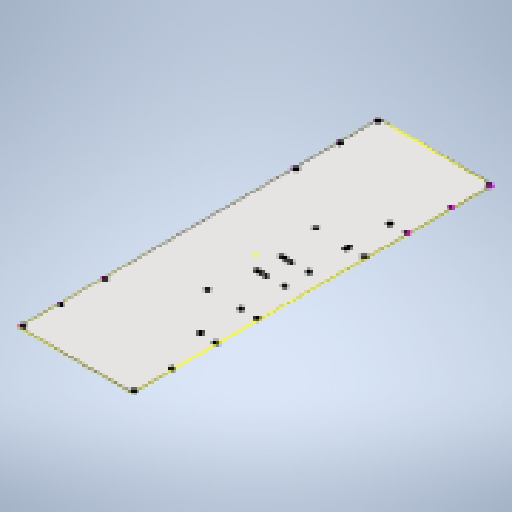
# Autodesk Inventor part: Base sheet2
Saved by Autodesk Inventor 2025.2 (Build 292293000, 293)
## iProperties
Created: 2025-05-26
Part Number: Base sheet2
Material: Generic
Document SubType Name: Sheet Metal
Designer: abdal
Density: 1 g/cm^3
Sheet Metal Rule: Default_mm
Appearance: Default
Author: abdal
Autodesk Inventor part; units mm, degrees
ref_plane "YZ Plane" through (0, 0, 0) normal (1, 0, 0) x (0, 1, 0)
ref_plane "XZ Plane" through (0, 0, 0) normal (0, 1, 0) x (-1, 0, 0)
ref_plane "XY Plane" through (0, 0, 0) normal (0, 0, 1) x (1, 0, 0)
sketch "Sketch1" plane through (0, 0, 0) normal (0, 1, 0) x (-1, 0, 0)
  line L0 (515, 1626) -> (-515, 1626)
  line L1 (-515, 1626) -> (-515, -1626)
  line L2 (-515, -1626) -> (515, -1626)
  line L3 (515, -1626) -> (515, 1626)
  line L4 (515, 1626) -> (-515, -1626) construction
  line L5 (-515, 1626) -> (515, -1626) construction
  point P0 (0, 0)
  dimension "d0" = 3252
  dimension "d1" = 1030
  measures "d0" distance of L2.end L0.start
  measures "d1" distance of L1.end L2.end
extrude "Plate1" add sketch "Sketch1" along normal blind 3
sketch "Sketch2" plane through (0, 0, 0) normal (0, -1, 0) x (1, 0, 0)
  line L0 (491, 1591.5799) -> (509, 1591.5799)
  ellipse E0 centre (509, 1594.777) end of major axis (509, 1597.9742) minor radius 3 (509, 1591.5799) -> (512, 1594.777) ccw
  line L1 (512, 1594.777) -> (512, 1613.9598)
  ellipse E1 centre (509, 1613.9598) end of major axis (509, 1610.7627) minor radius 3 (512, 1613.9598) -> (509, 1617.1569) ccw
  line L2 (509, 1617.1569) -> (491, 1617.1569)
  ellipse E2 centre (491, 1613.9598) end of major axis (491, 1610.7627) minor radius 3 (491, 1617.1569) -> (488, 1613.9598) ccw
  line L3 (488, 1613.9598) -> (488, 1594.777)
  ellipse E3 centre (491, 1594.777) end of major axis (491, 1597.9742) minor radius 3 (488, 1594.777) -> (491, 1591.5799) ccw
  line L4 (515, 1613.9598) -> (515, 1594.777)
  ellipse E4 centre (509, 1594.777) end of major axis (509, 1601.1713) minor radius 6 (509, 1588.3828) -> (515, 1594.777) ccw
  line L5 (509, 1588.3828) -> (491, 1588.3828)
  ellipse E5 centre (491, 1594.777) end of major axis (491, 1601.1713) minor radius 6 (485, 1594.777) -> (491, 1588.3828) ccw
  line L6 (485, 1594.777) -> (485, 1613.9598)
  ellipse E6 centre (491, 1613.9598) end of major axis (491, 1607.5655) minor radius 6 (491, 1620.354) -> (485, 1613.9598) ccw
  line L7 (491, 1620.354) -> (509, 1620.354)
  ellipse E7 centre (509, 1613.9598) end of major axis (509, 1607.5655) minor radius 6 (515, 1613.9598) -> (509, 1620.354) ccw
  line L8 (512, 1252) -> (512, 1270)
  arc A0 (512, 1270) -> (509, 1273) centre (509, 1270) ccw
  line L9 (509, 1273) -> (491, 1273)
  arc A1 (491, 1273) -> (488, 1270) centre (491, 1270) ccw
  line L10 (488, 1270) -> (488, 1252)
  arc A2 (488, 1252) -> (491, 1249) centre (491, 1252) ccw
  line L11 (491, 1249) -> (509, 1249)
  arc A3 (509, 1249) -> (512, 1252) centre (509, 1252) ccw
  line L12 (509, 1246) -> (491, 1246)
  arc A4 (485, 1252) -> (491, 1246) centre (491, 1252) ccw
  line L13 (485, 1252) -> (485, 1270)
  arc A5 (491, 1276) -> (485, 1270) centre (491, 1270) ccw
  line L14 (491, 1276) -> (509, 1276)
  arc A6 (515, 1270) -> (509, 1276) centre (509, 1270) ccw
  line L15 (515, 1270) -> (515, 1252)
  arc A7 (509, 1246) -> (515, 1252) centre (509, 1252) ccw
  line L16 (340.4848, 863.6493) -> (340.3575, 844.2981)
  ellipse E8 centre (343.3574, 844.2783) end of major axis (343.3787, 847.5035) minor radius 3 (340.3575, 844.2981) -> (343.3362, 841.0531) ccw
  line L17 (343.3362, 841.0531) -> (361.3358, 840.9347)
  ellipse E9 centre (361.3571, 844.1599) end of major axis (361.3783, 847.3851) minor radius 3 (361.3358, 840.9347) -> (364.357, 844.1401) ccw
  line L18 (364.357, 844.1401) -> (364.4843, 863.4914)
  ellipse E10 centre (361.4844, 863.5111) end of major axis (361.4632, 860.2859) minor radius 3 (364.4843, 863.4914) -> (361.5056, 866.7363) ccw
  line L19 (361.5056, 866.7363) -> (343.506, 866.8548)
  ellipse E11 centre (343.4848, 863.6296) end of major axis (343.4636, 860.4044) minor radius 3 (343.506, 866.8548) -> (340.4848, 863.6493) ccw
  ellipse E12 centre (343.4848, 863.6296) end of major axis (343.4423, 857.1792) minor radius 6 (343.5272, 870.08) -> (337.4849, 863.6691) ccw
  line L20 (343.5272, 870.08) -> (361.5268, 869.9616)
  ellipse E13 centre (361.4844, 863.5111) end of major axis (361.4419, 857.0607) minor radius 6 (367.4843, 863.4717) -> (361.5268, 869.9616) ccw
  line L21 (367.4843, 863.4717) -> (367.3569, 844.1204)
  ellipse E14 centre (361.3571, 844.1599) end of major axis (361.3995, 850.6103) minor radius 6 (361.3146, 837.7095) -> (367.3569, 844.1204) ccw
  line L22 (361.3146, 837.7095) -> (343.315, 837.8279)
  ellipse E15 centre (343.3574, 844.2783) end of major axis (343.3999, 850.7288) minor radius 6 (337.3576, 844.3178) -> (343.315, 837.8279) ccw
  line L23 (337.3576, 844.3178) -> (337.4849, 863.6691)
  line L24 (512, 852) -> (512, 870)
  arc A8 (512, 870) -> (509, 873) centre (509, 870) ccw
  line L25 (509, 873) -> (491, 873)
  arc A9 (491, 873) -> (488, 870) centre (491, 870) ccw
  line L26 (488, 870) -> (488, 852)
  arc A10 (488, 852) -> (491, 849) centre (491, 852) ccw
  line L27 (491, 849) -> (509, 849)
  arc A11 (509, 849) -> (512, 852) centre (509, 852) ccw
  line L28 (509, 846) -> (491, 846)
  arc A12 (485, 852) -> (491, 846) centre (491, 852) ccw
  line L29 (485, 852) -> (485, 870)
  arc A13 (491, 876) -> (485, 870) centre (491, 870) ccw
  line L30 (491, 876) -> (509, 876)
  arc A14 (515, 870) -> (509, 876) centre (509, 870) ccw
  line L31 (515, 870) -> (515, 852)
  arc A15 (509, 846) -> (515, 852) centre (509, 852) ccw
  line L32 (362, 477) -> (362, 495)
  arc A16 (362, 495) -> (359, 498) centre (359, 495) ccw
  line L33 (359, 498) -> (341, 498)
  arc A17 (341, 498) -> (338, 495) centre (341, 495) ccw
  line L34 (338, 495) -> (338, 477)
  arc A18 (338, 477) -> (341, 474) centre (341, 477) ccw
  line L35 (341, 474) -> (359, 474)
  arc A19 (359, 474) -> (362, 477) centre (359, 477) ccw
  line L36 (359, 471) -> (341, 471)
  arc A20 (335, 477) -> (341, 471) centre (341, 477) ccw
  line L37 (335, 477) -> (335, 495)
  arc A21 (341, 501) -> (335, 495) centre (341, 495) ccw
  line L38 (341, 501) -> (359, 501)
  arc A22 (365, 495) -> (359, 501) centre (359, 495) ccw
  line L39 (365, 495) -> (365, 477)
  arc A23 (359, 471) -> (365, 477) centre (359, 477) ccw
  line L40 (503.7539, 498) -> (484.8777, 498)
  ellipse E16 centre (484.8777, 495) end of major axis (488.0237, 495) minor radius 3 (484.8777, 498) -> (481.7317, 495) ccw
  line L41 (481.7317, 495) -> (481.7317, 477)
  ellipse E17 centre (484.8777, 477) end of major axis (488.0237, 477) minor radius 3 (481.7317, 477) -> (484.8777, 474) ccw
  line L42 (484.8777, 474) -> (503.7539, 474)
  ellipse E18 centre (503.7539, 477) end of major axis (500.6079, 477) minor radius 3 (503.7539, 474) -> (506.8999, 477) ccw
  line L43 (506.8999, 477) -> (506.8999, 495)
  ellipse E19 centre (503.7539, 495) end of major axis (500.6079, 495) minor radius 3 (506.8999, 495) -> (503.7539, 498) ccw
  ellipse E20 centre (503.7539, 477) end of major axis (497.4618, 477) minor radius 6 (503.7539, 471) -> (510.0459, 477) ccw
  line L44 (503.7539, 471) -> (484.8777, 471)
  ellipse E21 centre (484.8777, 477) end of major axis (491.1698, 477) minor radius 6 (478.5856, 477) -> (484.8777, 471) ccw
  line L45 (478.5856, 477) -> (478.5856, 495)
  ellipse E22 centre (484.8777, 495) end of major axis (491.1698, 495) minor radius 6 (484.8777, 501) -> (478.5856, 495) ccw
  line L46 (484.8777, 501) -> (503.7539, 501)
  ellipse E23 centre (503.7539, 495) end of major axis (497.4618, 495) minor radius 6 (510.0459, 495) -> (503.7539, 501) ccw
  line L47 (510.0459, 495) -> (510.0459, 477)
  line L48 (-515, 1626) -> (515, 1626) projected
  line L49 (515, 1626) -> (515, -1626) projected
  line L50 (515, -1626) -> (-515, -1626) projected
  line L51 (-515, -1626) -> (-515, 1626) projected
  line L52 (62.0059, 476.3985) -> (61.9941, 494.3985)
  ellipse E24 centre (58.9941, 494.3965) end of major axis (58.9961, 491.3965) minor radius 3 (61.9941, 494.3985) -> (58.9922, 497.3965) ccw
  line L53 (58.9922, 497.3965) -> (40.9922, 497.3847)
  ellipse E25 centre (40.9941, 494.3847) end of major axis (40.9961, 491.3847) minor radius 3 (40.9922, 497.3847) -> (37.9941, 494.3828) ccw
  line L54 (37.9941, 494.3828) -> (38.0059, 476.3828)
  ellipse E26 centre (41.0059, 476.3847) end of major axis (41.0039, 479.3847) minor radius 3 (38.0059, 476.3828) -> (41.0078, 473.3847) ccw
  line L55 (41.0078, 473.3847) -> (59.0078, 473.3965)
  ellipse E27 centre (59.0059, 476.3965) end of major axis (59.0039, 479.3965) minor radius 3 (59.0078, 473.3965) -> (62.0059, 476.3985) ccw
  ellipse E28 centre (59.0059, 476.3965) end of major axis (59.002, 482.3965) minor radius 6 (59.0098, 470.3965) -> (65.0059, 476.4004) ccw
  line L56 (59.0098, 470.3965) -> (41.0098, 470.3847)
  ellipse E29 centre (41.0059, 476.3847) end of major axis (41.002, 482.3847) minor radius 6 (35.0059, 476.3808) -> (41.0098, 470.3847) ccw
  line L57 (35.0059, 476.3808) -> (34.9941, 494.3808)
  ellipse E30 centre (40.9941, 494.3847) end of major axis (40.998, 488.3847) minor radius 6 (40.9902, 500.3847) -> (34.9941, 494.3808) ccw
  line L58 (40.9902, 500.3847) -> (58.9902, 500.3965)
  ellipse E31 centre (58.9941, 494.3965) end of major axis (58.998, 488.3965) minor radius 6 (64.9941, 494.4004) -> (58.9902, 500.3965) ccw
  line L59 (64.9941, 494.4004) -> (65.0059, 476.4004)
  line L60 (-509, 849) -> (-491, 849)
  arc A24 (-491, 849) -> (-488, 852) centre (-491, 852) ccw
  line L61 (-488, 852) -> (-488, 870)
  arc A25 (-488, 870) -> (-491, 873) centre (-491, 870) ccw
  line L62 (-491, 873) -> (-509, 873)
  arc A26 (-509, 873) -> (-512, 870) centre (-509, 870) ccw
  line L63 (-512, 870) -> (-512, 852)
  arc A27 (-512, 852) -> (-509, 849) centre (-509, 852) ccw
  line L64 (-485, 870) -> (-485, 852)
  arc A28 (-491, 846) -> (-485, 852) centre (-491, 852) ccw
  line L65 (-491, 846) -> (-509, 846)
  arc A29 (-515, 852) -> (-509, 846) centre (-509, 852) ccw
  line L66 (-515, 852) -> (-515, 870)
  arc A30 (-509, 876) -> (-515, 870) centre (-509, 870) ccw
  line L67 (-509, 876) -> (-491, 876)
  arc A31 (-485, 870) -> (-491, 876) centre (-491, 870) ccw
  line L68 (-488, 1252) -> (-488, 1270)
  arc A32 (-488, 1270) -> (-491, 1273) centre (-491, 1270) ccw
  line L69 (-491, 1273) -> (-509, 1273)
  arc A33 (-509, 1273) -> (-512, 1270) centre (-509, 1270) ccw
  line L70 (-512, 1270) -> (-512, 1252)
  arc A34 (-512, 1252) -> (-509, 1249) centre (-509, 1252) ccw
  line L71 (-509, 1249) -> (-491, 1249)
  arc A35 (-491, 1249) -> (-488, 1252) centre (-491, 1252) ccw
  line L72 (-491, 1246) -> (-509, 1246)
  arc A36 (-515, 1252) -> (-509, 1246) centre (-509, 1252) ccw
  line L73 (-515, 1252) -> (-515, 1270)
  arc A37 (-509, 1276) -> (-515, 1270) centre (-509, 1270) ccw
  line L74 (-509, 1276) -> (-491, 1276)
  arc A38 (-485, 1270) -> (-491, 1276) centre (-491, 1270) ccw
  line L75 (-485, 1270) -> (-485, 1252)
  arc A39 (-491, 1246) -> (-485, 1252) centre (-491, 1252) ccw
  line L76 (-509, 1591.5799) -> (-491, 1591.5799)
  ellipse E32 centre (-491, 1594.777) end of major axis (-491, 1597.9742) minor radius 3 (-491, 1591.5799) -> (-488, 1594.777) ccw
  line L77 (-488, 1594.777) -> (-488, 1613.9598)
  ellipse E33 centre (-491, 1613.9598) end of major axis (-491, 1610.7627) minor radius 3 (-488, 1613.9598) -> (-491, 1617.1569) ccw
  line L78 (-491, 1617.1569) -> (-509, 1617.1569)
  ellipse E34 centre (-509, 1613.9598) end of major axis (-509, 1610.7627) minor radius 3 (-509, 1617.1569) -> (-512, 1613.9598) ccw
  line L79 (-512, 1613.9598) -> (-512, 1594.777)
  ellipse E35 centre (-509, 1594.777) end of major axis (-509, 1597.9742) minor radius 3 (-512, 1594.777) -> (-509, 1591.5799) ccw
  line L80 (-485, 1613.9598) -> (-485, 1594.777)
  ellipse E36 centre (-491, 1594.777) end of major axis (-491, 1601.1713) minor radius 6 (-491, 1588.3828) -> (-485, 1594.777) ccw
  line L81 (-491, 1588.3828) -> (-509, 1588.3828)
  ellipse E37 centre (-509, 1594.777) end of major axis (-509, 1601.1713) minor radius 6 (-515, 1594.777) -> (-509, 1588.3828) ccw
  line L82 (-515, 1594.777) -> (-515, 1613.9598)
  ellipse E38 centre (-509, 1613.9598) end of major axis (-509, 1607.5655) minor radius 6 (-509, 1620.354) -> (-515, 1613.9598) ccw
  line L83 (-509, 1620.354) -> (-491, 1620.354)
  ellipse E39 centre (-491, 1613.9598) end of major axis (-491, 1607.5655) minor radius 6 (-485, 1613.9598) -> (-491, 1620.354) ccw
  line L84 (379, 123) -> (361, 123)
  arc A40 (361, 123) -> (358, 120) centre (361, 120) ccw
  line L85 (358, 120) -> (358, 102)
  arc A41 (358, 102) -> (361, 99) centre (361, 102) ccw
  line L86 (361, 99) -> (379, 99)
  arc A42 (379, 99) -> (382, 102) centre (379, 102) ccw
  line L87 (382, 102) -> (382, 120)
  arc A43 (382, 120) -> (379, 123) centre (379, 120) ccw
  line L88 (355, 102) -> (355, 120)
  arc A44 (361, 126) -> (355, 120) centre (361, 120) ccw
  line L89 (361, 126) -> (379, 126)
  arc A45 (385, 120) -> (379, 126) centre (379, 120) ccw
  line L90 (385, 120) -> (385, 102)
  arc A46 (379, 96) -> (385, 102) centre (379, 102) ccw
  line L91 (379, 96) -> (361, 96)
  arc A47 (355, 102) -> (361, 96) centre (361, 102) ccw
  ellipse E40 centre (144.9824, 120) end of major axis (163.6216, 120) minor radius 6 (144.9824, 126) -> (135, 125.067) ccw
  line L92 (144.9824, 126) -> (200.8999, 126)
  ellipse E41 centre (200.8999, 120) end of major axis (182.2608, 120) minor radius 6 (219.5391, 120) -> (200.8999, 126) ccw
  line L93 (219.5391, 120) -> (219.5391, 102)
  ellipse E42 centre (200.8999, 102) end of major axis (182.2608, 102) minor radius 6 (200.8999, 96) -> (219.5391, 102) ccw
  line L94 (200.8999, 96) -> (144.9824, 96)
  ellipse E43 centre (144.9824, 102) end of major axis (163.6216, 102) minor radius 6 (135, 96.933) -> (144.9824, 96) ccw
  line L95 (135, 96.933) -> (135, 125.067)
  ellipse E44 centre (144.9824, 102) end of major axis (154.302, 102) minor radius 3 (135.6628, 102) -> (144.9824, 99) ccw
  line L96 (144.9824, 99) -> (200.8999, 99)
  ellipse E45 centre (200.8999, 102) end of major axis (191.5803, 102) minor radius 3 (200.8999, 99) -> (210.2195, 102) ccw
  line L97 (210.2195, 102) -> (210.2195, 120)
  ellipse E46 centre (200.8999, 120) end of major axis (191.5803, 120) minor radius 3 (210.2195, 120) -> (200.8999, 123) ccw
  line L98 (200.8999, 123) -> (144.9824, 123)
  ellipse E47 centre (144.9824, 120) end of major axis (154.302, 120) minor radius 3 (144.9824, 123) -> (135.6628, 120) ccw
  line L99 (135.6628, 120) -> (135.6628, 102)
  line L100 (129, 123) -> (111, 123)
  arc A48 (111, 123) -> (108, 120) centre (111, 120) ccw
  line L101 (108, 120) -> (108, 102)
  arc A49 (108, 102) -> (111, 99) centre (111, 102) ccw
  line L102 (111, 99) -> (129, 99)
  arc A50 (129, 99) -> (132, 102) centre (129, 102) ccw
  line L103 (132, 102) -> (132, 120)
  arc A51 (132, 120) -> (129, 123) centre (129, 120) ccw
  line L104 (135, 120) -> (135, 102)
  arc A52 (129, 96) -> (135, 102) centre (129, 102) ccw
  line L105 (129, 96) -> (111, 96)
  arc A53 (105, 102) -> (111, 96) centre (111, 102) ccw
  line L106 (105, 102) -> (105, 120)
  arc A54 (111, 126) -> (105, 120) centre (111, 120) ccw
  line L107 (111, 126) -> (129, 126)
  arc A55 (135, 120) -> (129, 126) centre (129, 120) ccw
  line L108 (361, -123) -> (379, -123)
  arc A56 (379, -123) -> (382, -120) centre (379, -120) ccw
  line L109 (382, -120) -> (382, -102)
  arc A57 (382, -102) -> (379, -99) centre (379, -102) ccw
  line L110 (379, -99) -> (361, -99)
  arc A58 (361, -99) -> (358, -102) centre (361, -102) ccw
  line L111 (358, -102) -> (358, -120)
  arc A59 (358, -120) -> (361, -123) centre (361, -120) ccw
  line L112 (355, -120) -> (355, -102)
  arc A60 (361, -96) -> (355, -102) centre (361, -102) ccw
  line L113 (361, -96) -> (379, -96)
  arc A61 (385, -102) -> (379, -96) centre (379, -102) ccw
  line L114 (385, -102) -> (385, -120)
  arc A62 (379, -126) -> (385, -120) centre (379, -120) ccw
  line L115 (379, -126) -> (361, -126)
  arc A63 (355, -120) -> (361, -126) centre (361, -120) ccw
  line L116 (503.7539, -474) -> (484.8777, -474)
  ellipse E48 centre (484.8777, -477) end of major axis (488.0237, -477) minor radius 3 (484.8777, -474) -> (481.7317, -477) ccw
  line L117 (481.7317, -477) -> (481.7317, -495)
  ellipse E49 centre (484.8777, -495) end of major axis (488.0237, -495) minor radius 3 (481.7317, -495) -> (484.8777, -498) ccw
  line L118 (484.8777, -498) -> (503.7539, -498)
  ellipse E50 centre (503.7539, -495) end of major axis (500.6079, -495) minor radius 3 (503.7539, -498) -> (506.8999, -495) ccw
  line L119 (506.8999, -495) -> (506.8999, -477)
  ellipse E51 centre (503.7539, -477) end of major axis (500.6079, -477) minor radius 3 (506.8999, -477) -> (503.7539, -474) ccw
  ellipse E52 centre (503.7539, -495) end of major axis (497.4618, -495) minor radius 6 (503.7539, -501) -> (510.0459, -495) ccw
  line L120 (503.7539, -501) -> (484.8777, -501)
  ellipse E53 centre (484.8777, -495) end of major axis (491.1698, -495) minor radius 6 (478.5856, -495) -> (484.8777, -501) ccw
  line L121 (478.5856, -495) -> (478.5856, -477)
  ellipse E54 centre (484.8777, -477) end of major axis (491.1698, -477) minor radius 6 (484.8777, -471) -> (478.5856, -477) ccw
  line L122 (484.8777, -471) -> (503.7539, -471)
  ellipse E55 centre (503.7539, -477) end of major axis (497.4618, -477) minor radius 6 (510.0459, -477) -> (503.7539, -471) ccw
  line L123 (510.0459, -477) -> (510.0459, -495)
  line L124 (362, -495) -> (362, -477)
  arc A64 (362, -477) -> (359, -474) centre (359, -477) ccw
  line L125 (359, -474) -> (341, -474)
  arc A65 (341, -474) -> (338, -477) centre (341, -477) ccw
  line L126 (338, -477) -> (338, -495)
  arc A66 (338, -495) -> (341, -498) centre (341, -495) ccw
  line L127 (341, -498) -> (359, -498)
  arc A67 (359, -498) -> (362, -495) centre (359, -495) ccw
  line L128 (359, -501) -> (341, -501)
  arc A68 (335, -495) -> (341, -501) centre (341, -495) ccw
  line L129 (335, -495) -> (335, -477)
  arc A69 (341, -471) -> (335, -477) centre (341, -477) ccw
  line L130 (341, -471) -> (359, -471)
  arc A70 (365, -477) -> (359, -471) centre (359, -477) ccw
  line L131 (365, -477) -> (365, -495)
  arc A71 (359, -501) -> (365, -495) centre (359, -495) ccw
  ellipse E56 centre (341, -454.707) end of major axis (341, -463.2911) minor radius 6 (341, -446.1229) -> (335, -454.707) ccw
  line L132 (341, -446.1229) -> (359, -446.1229)
  ellipse E57 centre (359, -454.707) end of major axis (359, -463.2911) minor radius 6 (365, -454.707) -> (359, -446.1229) ccw
  line L133 (365, -454.707) -> (365, -471)
  line L134 (365, -471) -> (362, -471)
  line L135 (362, -471) -> (362, -454.707)
  ellipse E58 centre (359, -454.707) end of major axis (359, -458.9991) minor radius 3 (362, -454.707) -> (359, -450.415) ccw
  line L136 (359, -450.415) -> (341, -450.415)
  ellipse E59 centre (341, -454.707) end of major axis (341, -458.9991) minor radius 3 (341, -450.415) -> (338, -454.707) ccw
  line L137 (338, -454.707) -> (338, -471)
  line L138 (338, -471) -> (335, -471)
  line L139 (335, -471) -> (335, -454.707)
  line L140 (62, -495) -> (62, -477)
  arc A72 (62, -477) -> (59, -474) centre (59, -477) ccw
  line L141 (59, -474) -> (41, -474)
  arc A73 (41, -474) -> (38, -477) centre (41, -477) ccw
  line L142 (38, -477) -> (38, -495)
  arc A74 (38, -495) -> (41, -498) centre (41, -495) ccw
  line L143 (41, -498) -> (59, -498)
  arc A75 (59, -498) -> (62, -495) centre (59, -495) ccw
  line L144 (41, -471) -> (59, -471)
  arc A76 (65, -477) -> (59, -471) centre (59, -477) ccw
  line L145 (65, -477) -> (65, -495)
  arc A77 (59, -501) -> (65, -495) centre (59, -495) ccw
  line L146 (59, -501) -> (41, -501)
  arc A78 (35, -495) -> (41, -501) centre (41, -495) ccw
  line L147 (35, -495) -> (35, -477)
  arc A79 (41, -471) -> (35, -477) centre (41, -477) ccw
  line L148 (364.529, -863.49) -> (364.3993, -844.1387)
  ellipse E60 centre (361.3994, -844.1588) end of major axis (361.421, -847.384) minor radius 3 (364.3993, -844.1387) -> (361.3778, -840.9336) ccw
  line L149 (361.3778, -840.9336) -> (343.3782, -841.0542)
  ellipse E61 centre (343.3998, -844.2794) end of major axis (343.4214, -847.5046) minor radius 3 (343.3782, -841.0542) -> (340.3999, -844.2995) ccw
  line L150 (340.3999, -844.2995) -> (340.5295, -863.6507)
  ellipse E62 centre (343.5294, -863.6306) end of major axis (343.5078, -860.4054) minor radius 3 (340.5295, -863.6507) -> (343.551, -866.8558) ccw
  line L151 (343.551, -866.8558) -> (361.5506, -866.7353)
  ellipse E63 centre (361.529, -863.5101) end of major axis (361.5074, -860.2849) minor radius 3 (361.5506, -866.7353) -> (364.529, -863.49) ccw
  ellipse E64 centre (361.529, -863.5101) end of major axis (361.4858, -857.0597) minor radius 6 (361.5722, -869.9605) -> (367.5289, -863.4699) ccw
  line L152 (361.5722, -869.9605) -> (343.5726, -870.0811)
  ellipse E65 centre (343.5294, -863.6306) end of major axis (343.4862, -857.1802) minor radius 6 (337.5296, -863.6708) -> (343.5726, -870.0811) ccw
  line L153 (337.5296, -863.6708) -> (337.3999, -844.3196)
  ellipse E66 centre (343.3998, -844.2794) end of major axis (343.443, -850.7298) minor radius 6 (343.3566, -837.829) -> (337.3999, -844.3196) ccw
  line L154 (343.3566, -837.829) -> (361.3562, -837.7084)
  ellipse E67 centre (361.3994, -844.1588) end of major axis (361.4426, -850.6092) minor radius 6 (367.3993, -844.1186) -> (361.3562, -837.7084) ccw
  line L155 (367.3993, -844.1186) -> (367.5289, -863.4699)
  line L156 (488, -852) -> (488, -870)
  arc A80 (488, -870) -> (491, -873) centre (491, -870) ccw
  line L157 (491, -873) -> (509, -873)
  arc A81 (509, -873) -> (512, -870) centre (509, -870) ccw
  line L158 (512, -870) -> (512, -852)
  arc A82 (512, -852) -> (509, -849) centre (509, -852) ccw
  line L159 (509, -849) -> (491, -849)
  arc A83 (491, -849) -> (488, -852) centre (491, -852) ccw
  line L160 (509, -876) -> (491, -876)
  arc A84 (485, -870) -> (491, -876) centre (491, -870) ccw
  line L161 (485, -870) -> (485, -852)
  arc A85 (491, -846) -> (485, -852) centre (491, -852) ccw
  line L162 (491, -846) -> (509, -846)
  arc A86 (515, -852) -> (509, -846) centre (509, -852) ccw
  line L163 (515, -852) -> (515, -870)
  arc A87 (509, -876) -> (515, -870) centre (509, -870) ccw
  line L164 (488, -1252) -> (488, -1270)
  arc A88 (488, -1270) -> (491, -1273) centre (491, -1270) ccw
  line L165 (491, -1273) -> (509, -1273)
  arc A89 (509, -1273) -> (512, -1270) centre (509, -1270) ccw
  line L166 (512, -1270) -> (512, -1252)
  arc A90 (512, -1252) -> (509, -1249) centre (509, -1252) ccw
  line L167 (509, -1249) -> (491, -1249)
  arc A91 (491, -1249) -> (488, -1252) centre (491, -1252) ccw
  line L168 (509, -1276) -> (491, -1276)
  arc A92 (485, -1270) -> (491, -1276) centre (491, -1270) ccw
  line L169 (485, -1270) -> (485, -1252)
  arc A93 (491, -1246) -> (485, -1252) centre (491, -1252) ccw
  line L170 (491, -1246) -> (509, -1246)
  arc A94 (515, -1252) -> (509, -1246) centre (509, -1252) ccw
  line L171 (515, -1252) -> (515, -1270)
  arc A95 (509, -1276) -> (515, -1270) centre (509, -1270) ccw
  line L172 (512, -1613.9598) -> (512, -1594.777)
  ellipse E68 centre (509, -1594.777) end of major axis (509, -1597.9742) minor radius 3 (512, -1594.777) -> (509, -1591.5799) ccw
  line L173 (509, -1591.5799) -> (491, -1591.5799)
  ellipse E69 centre (491, -1594.777) end of major axis (491, -1597.9742) minor radius 3 (491, -1591.5799) -> (488, -1594.777) ccw
  line L174 (488, -1594.777) -> (488, -1613.9598)
  ellipse E70 centre (491, -1613.9598) end of major axis (491, -1610.7627) minor radius 3 (488, -1613.9598) -> (491, -1617.1569) ccw
  line L175 (491, -1617.1569) -> (509, -1617.1569)
  ellipse E71 centre (509, -1613.9598) end of major axis (509, -1610.7627) minor radius 3 (509, -1617.1569) -> (512, -1613.9598) ccw
  line L176 (485, -1613.9598) -> (485, -1594.777)
  ellipse E72 centre (491, -1594.777) end of major axis (491, -1601.1713) minor radius 6 (491, -1588.3828) -> (485, -1594.777) ccw
  line L177 (491, -1588.3828) -> (509, -1588.3828)
  ellipse E73 centre (509, -1594.777) end of major axis (509, -1601.1713) minor radius 6 (515, -1594.777) -> (509, -1588.3828) ccw
  line L178 (515, -1594.777) -> (515, -1613.9598)
  ellipse E74 centre (509, -1613.9598) end of major axis (509, -1607.5655) minor radius 6 (509, -1620.354) -> (515, -1613.9598) ccw
  line L179 (509, -1620.354) -> (491, -1620.354)
  ellipse E75 centre (491, -1613.9598) end of major axis (491, -1607.5655) minor radius 6 (485, -1613.9598) -> (491, -1620.354) ccw
  line L180 (-491, -1591.5799) -> (-509, -1591.5799)
  ellipse E76 centre (-509, -1594.777) end of major axis (-509, -1597.9742) minor radius 3 (-509, -1591.5799) -> (-512, -1594.777) ccw
  line L181 (-512, -1594.777) -> (-512, -1613.9598)
  ellipse E77 centre (-509, -1613.9598) end of major axis (-509, -1610.7627) minor radius 3 (-512, -1613.9598) -> (-509, -1617.1569) ccw
  line L182 (-509, -1617.1569) -> (-491, -1617.1569)
  ellipse E78 centre (-491, -1613.9598) end of major axis (-491, -1610.7627) minor radius 3 (-491, -1617.1569) -> (-488, -1613.9598) ccw
  line L183 (-488, -1613.9598) -> (-488, -1594.777)
  ellipse E79 centre (-491, -1594.777) end of major axis (-491, -1597.9742) minor radius 3 (-488, -1594.777) -> (-491, -1591.5799) ccw
  line L184 (-515, -1613.9598) -> (-515, -1594.777)
  ellipse E80 centre (-509, -1594.777) end of major axis (-509, -1601.1713) minor radius 6 (-509, -1588.3828) -> (-515, -1594.777) ccw
  line L185 (-509, -1588.3828) -> (-491, -1588.3828)
  ellipse E81 centre (-491, -1594.777) end of major axis (-491, -1601.1713) minor radius 6 (-485, -1594.777) -> (-491, -1588.3828) ccw
  line L186 (-485, -1594.777) -> (-485, -1613.9598)
  ellipse E82 centre (-491, -1613.9598) end of major axis (-491, -1607.5655) minor radius 6 (-491, -1620.354) -> (-485, -1613.9598) ccw
  line L187 (-491, -1620.354) -> (-509, -1620.354)
  ellipse E83 centre (-509, -1613.9598) end of major axis (-509, -1607.5655) minor radius 6 (-515, -1613.9598) -> (-509, -1620.354) ccw
  line L188 (-512, -1252) -> (-512, -1270)
  arc A96 (-512, -1270) -> (-509, -1273) centre (-509, -1270) ccw
  line L189 (-509, -1273) -> (-491, -1273)
  arc A97 (-491, -1273) -> (-488, -1270) centre (-491, -1270) ccw
  line L190 (-488, -1270) -> (-488, -1252)
  arc A98 (-488, -1252) -> (-491, -1249) centre (-491, -1252) ccw
  line L191 (-491, -1249) -> (-509, -1249)
  arc A99 (-509, -1249) -> (-512, -1252) centre (-509, -1252) ccw
  line L192 (-491, -1276) -> (-509, -1276)
  arc A100 (-515, -1270) -> (-509, -1276) centre (-509, -1270) ccw
  line L193 (-515, -1270) -> (-515, -1252)
  arc A101 (-509, -1246) -> (-515, -1252) centre (-509, -1252) ccw
  line L194 (-509, -1246) -> (-491, -1246)
  arc A102 (-485, -1252) -> (-491, -1246) centre (-491, -1252) ccw
  line L195 (-485, -1252) -> (-485, -1270)
  arc A103 (-491, -1276) -> (-485, -1270) centre (-491, -1270) ccw
  line L196 (-509, -873) -> (-491, -873)
  arc A104 (-491, -873) -> (-488, -870) centre (-491, -870) ccw
  line L197 (-488, -870) -> (-488, -852)
  arc A105 (-488, -852) -> (-491, -849) centre (-491, -852) ccw
  line L198 (-491, -849) -> (-509, -849)
  arc A106 (-509, -849) -> (-512, -852) centre (-509, -852) ccw
  line L199 (-512, -852) -> (-512, -870)
  arc A107 (-512, -870) -> (-509, -873) centre (-509, -870) ccw
  line L200 (-485, -852) -> (-485, -870)
  arc A108 (-491, -876) -> (-485, -870) centre (-491, -870) ccw
  line L201 (-491, -876) -> (-509, -876)
  arc A109 (-515, -870) -> (-509, -876) centre (-509, -870) ccw
  line L202 (-515, -870) -> (-515, -852)
  arc A110 (-509, -846) -> (-515, -852) centre (-509, -852) ccw
  line L203 (-509, -846) -> (-491, -846)
  arc A111 (-485, -852) -> (-491, -846) centre (-491, -852) ccw
  line L204 (132, -120) -> (132, -102)
  arc A112 (132, -102) -> (129, -99) centre (129, -102) ccw
  line L205 (129, -99) -> (111, -99)
  arc A113 (111, -99) -> (108, -102) centre (111, -102) ccw
  line L206 (108, -102) -> (108, -120)
  arc A114 (108, -120) -> (111, -123) centre (111, -120) ccw
  line L207 (111, -123) -> (129, -123)
  arc A115 (129, -123) -> (132, -120) centre (129, -120) ccw
  line L208 (129, -126) -> (111, -126)
  arc A116 (105, -120) -> (111, -126) centre (111, -120) ccw
  line L209 (105, -120) -> (105, -102)
  arc A117 (111, -96) -> (105, -102) centre (111, -102) ccw
  line L210 (111, -96) -> (129, -96)
  arc A118 (135, -102) -> (129, -96) centre (129, -102) ccw
  line L211 (135, -102) -> (135, -120)
  arc A119 (129, -126) -> (135, -120) centre (129, -120) ccw
  ellipse E84 centre (144.9751, -102) end of major axis (163.6148, -102) minor radius 6 (144.9751, -96) -> (135, -96.9315) ccw
  line L212 (144.9751, -96) -> (200.8943, -96)
  ellipse E85 centre (200.8943, -102) end of major axis (182.2545, -102) minor radius 6 (219.534, -102) -> (200.8943, -96) ccw
  line L213 (219.534, -102) -> (219.534, -120)
  ellipse E86 centre (200.8943, -120) end of major axis (182.2545, -120) minor radius 6 (200.8943, -126) -> (219.534, -120) ccw
  line L214 (200.8943, -126) -> (144.9751, -126)
  ellipse E87 centre (144.9751, -120) end of major axis (163.6148, -120) minor radius 6 (135, -125.0685) -> (144.9751, -126) ccw
  line L215 (135, -125.0685) -> (135, -96.9315)
  ellipse E88 centre (144.9751, -120) end of major axis (154.295, -120) minor radius 3 (135.6552, -120) -> (144.9751, -123) ccw
  line L216 (144.9751, -123) -> (200.8943, -123)
  ellipse E89 centre (200.8943, -120) end of major axis (191.5744, -120) minor radius 3 (200.8943, -123) -> (210.2141, -120) ccw
  line L217 (210.2141, -120) -> (210.2141, -102)
  ellipse E90 centre (200.8943, -102) end of major axis (191.5744, -102) minor radius 3 (210.2141, -102) -> (200.8943, -99) ccw
  line L218 (200.8943, -99) -> (144.9751, -99)
  ellipse E91 centre (144.9751, -102) end of major axis (154.295, -102) minor radius 3 (144.9751, -99) -> (135.6552, -102) ccw
  line L219 (135.6552, -102) -> (135.6552, -120)
  point P0 (0, 0)
  constraints: 432 end point, 240 point on circle, 120 centre point, 92 horizontal, 92 vertical, 1162 other
extrude "Extrusion1" cut sketch "Sketch2" against normal through all contours E3 L3 E2 L2 E1 L1 E0 L0 | L4 E4 L5 E5 L6 E6 L7 E7 | L15 A7 L12 A4 L13 A5 L14 A6 | E38 L83 E39 L80 E36 L81 E37 L51 | L31 A15 L28 A12 L29 A13 L30 A14 | A37 L74 A38 L75 A39 L72 A36 L51 | L49 A87 L160 A84 L161 A85 L162 A86 | A30 L67 A31 L64 A28 L65 A29 L51 | L49 A95 L168 A92 L169 A93 L170 A94 | A110 L203 A111 L200 A108 L201 A109 L51 | L49 E74 L179 E75 L176 E72 L177 E73 | A101 L194 A102 L195 A103 L192 A100 L51 | E80 L185 E81 L186 E82 L187 E83 L51 | A3 L11 A2 L10 A1 L9 A0 L8 | E11 L19 E10 L18 E9 L17 E8 L16 | L20 E13 L21 E14 L22 E15 L23 E12 | A11 L27 A10 L26 A9 L25 A8 L24 | A19 L35 A18 L34 A17 L33 A16 L32 | L36 A20 L37 A21 L38 A22 L39 A23 | E19 L43 E18 L42 E17 L41 E16 L40 | L44 E21 L45 E22 L46 E23 L47 E20 | E27 L55 E26 L54 E25 L53 E24 L52 | L56 E29 L57 E30 L58 E31 L59 E28 | A27 L63 A26 L62 A25 L61 A24 L60 | A35 L71 A34 L70 A33 L69 A32 L68 | E35 L79 E34 L78 E33 L77 E32 L76 | A43 L87 A42 L86 A41 L85 A40 L84 | L88 A44 L89 A45 L90 A46 L91 A47 | L92 E41 L93 E42 L94 E43 L95 E40 | L95 A52 L105 A53 L106 A54 L107 A55 | L99 E47 L98 E46 L97 E45 L96 E44 | A51 L103 A50 L102 A49 L101 A48 L100 | A59 L111 A58 L110 A57 L109 A56 L108 | L112 A60 L113 A61 L114 A62 L115 A63 | E51 L119 E50 L118 E49 L117 E48 L116 | L120 E53 L121 E54 L122 E55 L123 E52 | A67 L127 A66 L126 A65 L125 A64 L124 | L128 A68 L129 A69 L130 A70 L131 A71 | L132 E57 L133 L134 L135 E58 L136 E59 L137 L138 L139 E56 | A75 L143 A74 L142 A73 L141 A72 L140 | L144 A76 L145 A77 L146 A78 L147 A79 | E63 L151 E62 L150 E61 L149 E60 L148 | L152 E65 L153 E66 L154 E67 L155 E64 | A83 L159 A82 L158 A81 L157 A80 L156 | A91 L167 A90 L166 A89 L165 A88 L164 | E71 L175 E70 L174 E69 L173 E68 L172 | E79 L183 E78 L182 E77 L181 E76 L180 | A99 L191 A98 L190 A97 L189 A96 L188 | A107 L199 A106 L198 A105 L197 A104 L196 | A115 L207 A114 L206 A113 L205 A112 L204 | L208 A116 L209 A117 L210 A118 L211 A119 | L211 L215 E84 L212 E85 L213 E86 L214 E87 | L219 E91 L218 E90 L217 E89 L216 E88
sketch "Sketch3" plane through (0, 0, 0) normal (0, -1, 0) x (1, 0, 0)
  line L0 (365, -477) -> (365, -495) projected
  line L1 (335, -454.707) -> (365, -454.707)
  line L2 (365, -454.707) -> (365, -487.293)
  line L3 (365, -487.293) -> (335, -487.293)
  line L4 (335, -487.293) -> (335, -454.707)
  line L5 (359, -471) -> (341, -471) projected
  line L6 (335, -454.707) -> (365, -487.293) construction
  line L7 (365, -454.707) -> (335, -487.293) construction
  ellipse E0 centre (359, -454.707) end of major axis (359, -463.2911) minor radius 6 (365, -454.707) -> (359, -446.1229) ccw projected
  line L8 (362.8222, -454.707) -> (337.2898, -454.707)
  line L9 (337.2898, -454.707) -> (337.2898, -449.941)
  line L10 (337.2898, -449.941) -> (362.8222, -449.941)
  line L11 (362.8222, -449.941) -> (362.8222, -454.707)
  point P0 (0, 0)
  point P1 (350, -471)
  constraints: 20 end point, 4 parallel, 3 midpoint, 2 horizontal, 2 perpendicular, 2 point on line, 2 other
extrude "Extrusion2" cut sketch "Sketch3" against normal through all
equation "\"d2\" = Thickness"
equation "\"BendRadius\" = Thickness"
equation "\"BendReliefWidth\" = Thickness"
equation "\"BendReliefDepth\" = 0.5 * Thickness"
equation "\"CornerReliefSize\" = 4 * Thickness"
equation "\"MinimumRemnant\" = 2 * Thickness"
equation "\"TransitionRadius\" = BendRadius"
equation "\"JacobiRadiusSize\" = BendRadius"
equation "\"GapSize\" = Thickness"
equation "\"Thickness\" = 3"
body "Solid1"
